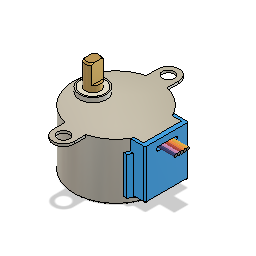
28BYJ-48 (Autodesk Fusion 360 design; units mm, degrees)
Autodesk Fusion 360 part; units mm, degrees
sketch "Sketch1" plane through (0, 0, 0) normal (0, 1, 0) x (1, 0, 0)
  circle A0 centre (0, 0) radius 14
  dimension "d1" = 28
  constraint coincident A0.centre origin
  measures "d1" diameter of A0
extrude "Extrude1" add sketch "Sketch1" along normal blind 19 makes body 1
sketch "Sketch2" plane through (0, 19, 0) normal (0, 1, 0) x (-1, 0, 0)
  circle A0 centre (0, 0) radius 14
  line L0 (14, 0) -> (-15.5, 0)
  line L1 (-15.5, 0) -> (-15.5, -6.3)
  line L2 (-15.5, -6.3) -> (-12.5024, -6.3)
  line L3 (-15.5, 0) -> (-15.5, 6.3)
  line L4 (-15.5, 6.3) -> (-12.5024, 6.3)
  dimension "d4" = 29.5
  dimension "d5" = 6.3
  dimension "d6" = 6.3
  constraint coincident A0 L0.start
  constraint horizontal L0
  constraint perpendicular L0 L1
  constraint coincident A0 L2.end
  constraint perpendicular L1 L2
  constraint perpendicular L0 L3
  constraint coincident A0 L4.end
  constraint perpendicular L3 L4
  measures "d4" distance of L0.start L0.end
  measures "d5" distance of L0.end L1.end
  measures "d6" distance of L0.end L3.end
extrude "Extrude2" add sketch "Sketch2" against normal blind 10 contours A0 L0 L3 L4 | A0 L0 L1 L2 bodies 1
sketch "Sketch3" plane through (0, 19, 0) normal (0, 1, 0) x (-1, 0, 0)
  arc A0 (-12.5024, -6.3) -> (-12.5024, 6.3) centre (0, 0) ccw
  line L0 (-12.5024, 6.3) -> (-15.5, 6.3)
  line L1 (-15.5, 6.3) -> (-15.5, -6.3)
  line L2 (-15.5, -6.3) -> (-12.5024, -6.3)
  line L3 (14, 0) -> (3.2, 0)
  circle A1 centre (7.7, 0) radius 4.5
  circle A2 centre (7.7, 0) radius 4
  dimension "d9" = 10.8
  dimension "d11" = 9
  dimension "d12" = 8
  constraint midpoint A0 L3.start
  constraint horizontal L3
  constraint coincident L3.end A1
  constraint concentric A1 A2
  measures "d9" distance of L3.start L3.end
  measures "d11" diameter of A1
  measures "d12" diameter of A2
extrude "Extrude3" add sketch "Sketch3" along normal blind 1.5 contours L3 A1 A2 | L3 A1 A2 bodies 1
sketch "Sketch4" plane through (0, 19, 0) normal (0, 1, 0) x (-1, 0, 0)
  circle A0 centre (7.7, 0) radius 4
  circle A1 centre (7.7, 0) radius 4
  circle A2 centre (7.7, 0) radius 2.5
  dimension "d15" = 5
  constraint concentric A0 A1
  constraint concentric A1 A2
  measures "d15" diameter of A2
extrude "Extrude4" add sketch "Sketch4" along normal blind 1.5 separate body makes body 2
sketch "Sketch5" plane through (0, 19, 0) normal (0, 1, 0) x (-1, 0, 0)
  circle A0 centre (7.7, 0) radius 4
  circle A1 centre (7.7, 0) radius 2.5
  dimension "d18" = 5
  constraint concentric A0 A1
  measures "d18" diameter of A1
extrude "Extrude5" cut sketch "Sketch5" against normal blind 15 contours A1 bodies 1
extrude "Extrude6" add 1 faces at (-8.3885, 4, -0.2537) along direction (0, 1, 0) blind 24.75 separate body on bodies 1 makes body 3
sketch "Sketch6" plane through (0, 28.75, 0) normal (0, 1, 0) x (-1, 0, 0)
  circle A0 centre (7.7, 0) radius 2.5
  circle A1 centre (7.7, 0) radius 1.5
  line L0 (9.2, 0) -> (9.2, -2)
  line L1 (6.2, 0) -> (6.2, -2)
  line L2 (9.2, 0) -> (9.2, 2)
  line L3 (6.2, 0) -> (6.2, 2)
  dimension "d23" = 3
  constraint concentric A0 A1
  constraint coincident A1 L0.start
  constraint coincident A0 L0.end
  constraint tangent A1 L0
  constraint vertical L0
  constraint coincident A1 L1.start
  constraint coincident A0 L1.end
  constraint tangent A1 L1
  constraint parallel L0 L1
  constraint coincident A0 L2.end
  constraint tangent A1 L2
  constraint coincident A0 L3.end
  constraint tangent A1 L3
  measures "d23" diameter of A1
extrude "Extrude7" cut sketch "Sketch6" against normal blind 6.25 contours A0 L0 L2 | A0 L1 L3 bodies 3
chamfer "Chamfer1" distance 0.5 angle 45 2 edges at (-7.7, 28.75, 2.5) (-7.7, 28.75, -2.5) on bodies 3
sketch "Sketch7" plane through (0, 19, 0) normal (0, 1, 0) x (-1, 0, 0)
  arc A0 (-12.5024, -6.3) -> (-12.5024, 6.3) centre (0, 0) ccw
  line L0 (-12.5024, 6.3) -> (-15.5, 6.3)
  line L1 (-15.5, 6.3) -> (-15.5, -6.3)
  line L2 (-15.5, -6.3) -> (-12.5024, -6.3)
  circle A1 centre (7.7, 0) radius 4.5
  circle A2 centre (0, -17.5) radius 2
  circle A3 centre (0, 17.5) radius 2
  arc A4 (-3.5, -17.5) -> (3.5, -17.5) centre (0, -17.5) ccw
  arc A5 (3.5, 17.5) -> (-3.5, 17.5) centre (0, 17.5) ccw
  line L3 (3.5, -17.5) -> (3.5, -13.5554)
  line L4 (-3.5, -17.5) -> (-3.5, -13.5554)
  line L5 (-3.5, 13.5554) -> (-3.5, 17.5)
  arc A6 (3.5, 13.5554) -> (-3.5, 13.5554) centre (0, 0) ccw
  arc A7 (-3.5, -13.5554) -> (3.5, -13.5554) centre (0, 0) ccw
  line L6 (3.5, 13.5554) -> (3.5, 17.5)
  dimension "d27" = 17.5
  dimension "d28" = 17.5
  dimension "d29" = 4
  dimension "d30" = 4
  dimension "d31" = 7
  dimension "d32" = 7
  constraint concentric A2 A4
  constraint concentric A3 A5
  constraint tangent A5 L3
  constraint vertical L3
  constraint tangent A5 L4
  constraint vertical L4
  constraint coincident A0.centre A6.centre
  constraint coincident A6.start L3
  constraint coincident A0 L4.end
  constraint coincident A0 L5.start
  constraint collinear L4 L5
  constraint concentric A6 A7
  measures "d27" distance of A0.centre A2.centre
  measures "d28" distance of A0.centre A3.centre
  measures "d29" diameter of A2
  measures "d30" diameter of A3
  measures "d31" diameter of A4
  measures "d32" diameter of A5
extrude "Extrude8" add sketch "Sketch7" against normal blind 0.8 contours A0 A4 L3 L4 A7 | A0 A5 L5 A6 L6 bodies 1
fillet "Fillet1" radius 0.5 1 edges at (-13.0526, 0, 5.0626) on bodies 1
sketch "Sketch8" plane through (0, 19, 0) normal (0, 1, 0) x (-1, 0, 0)
  circle A0 centre (0, -17.5) radius 2
  circle A1 centre (0, 17.5) radius 2
  arc A2 (-12.5024, -6.3) -> (-3.5, -13.5554) centre (0, 0) ccw
  line L0 (-3.5, -13.5554) -> (-3.5, -17.5)
  arc A3 (-3.5, -17.5) -> (3.5, -17.5) centre (0, -17.5) ccw
  line L1 (3.5, -17.5) -> (3.5, -13.5554)
  arc A4 (3.5, -13.5554) -> (3.5, 13.5554) centre (0, 0) ccw
  line L2 (3.5, 13.5554) -> (3.5, 17.5)
  arc A5 (3.5, 17.5) -> (-3.5, 17.5) centre (0, 17.5) ccw
  line L3 (-3.5, 17.5) -> (-3.5, 13.5554)
  arc A6 (-3.5, 13.5554) -> (-12.5024, 6.3) centre (0, 0) ccw
  line L4 (-12.5024, 6.3) -> (-15.5, 6.3)
  line L5 (-15.5, 6.3) -> (-15.5, -6.3)
  line L6 (-15.5, -6.3) -> (-12.5024, -6.3)
  circle A7 centre (7.7, 0) radius 4.5
  line L7 (14, 0) -> (-17, 0)
  line L8 (-17, 0) -> (-17, -7.25)
  line L9 (-17, -7.25) -> (-11.9765, -7.25)
  line L10 (-17, 0) -> (-17, 7.25)
  line L11 (-17, 7.25) -> (-11.9765, 7.25)
  dimension "d37" = 7.25
  dimension "d38" = 7.25
  constraint midpoint A4 L7.start
  constraint horizontal L7
  constraint perpendicular L7 L8
  constraint coincident A2 L9.end
  constraint perpendicular L8 L9
  constraint perpendicular L7 L10
  constraint coincident A6 L11.end
  constraint perpendicular L10 L11
  measures "d37" distance of L7.end L8.end
  measures "d38" distance of L7.end L10.end
extrude "Extrude9" add sketch "Sketch8" against normal blind 16.5 separate body contours A2 L5 L6 L7 L8 L9 | A6 L4 L5 L7 L10 L11 makes body 4
sketch "Sketch9" plane through (0, 9, 0) normal (0, -1, 0) x (1, 0, 0)
  line L0 (15.5, -6.3) -> (15.5, 6.3)
  line L1 (15.5, 6.3) -> (12.5024, 6.3)
  arc A0 (12.5024, -6.3) -> (12.5024, 6.3) centre (0, 0) ccw
  line L2 (12.5024, -6.3) -> (15.5, -6.3)
extrude "Extrude10" add sketch "Sketch9" along normal blind 6.5 bodies 4
ref_plane "WorkPlane1" through (14.4883, 15.2, 0) normal (0, 1, 0) x (-1, 0, 0)
sketch "Sketch10" plane through (14.4883, 15.2, 0) normal (0, 1, 0) x (1, 0, 0)
  line L0 (-14.5, 17.5) -> (-14.5, -17.5)
  circle A0 centre (-14.5, 0) radius 15
  line L1 (-14.5, 0) -> (-14.5, 8.625)
  line L2 (-14.5, 8.625) -> (-2.2277, 8.625)
  line L3 (-14.5, 0) -> (-14.5, -8.625)
  line L4 (-14.5, -8.625) -> (-2.2277, -8.625)
  circle A1 centre (-14.5, 0) radius 14
  dimension "d44" = 30
  dimension "d45" = 8.625
  dimension "d46" = 8.625
  dimension "d47" = 28
  constraint vertical L0
  constraint midpoint L0 A0.centre
  constraint coincident A0.centre L1.start
  constraint parallel L0 L1
  constraint coincident A0 L2.end
  constraint perpendicular L1 L2
  constraint perpendicular L2 L3
  constraint coincident A0 L4.end
  constraint perpendicular L0 L4
  constraint concentric A0 A1
  measures "d44" diameter of A0
  measures "d45" distance of A0.centre L1.end
  measures "d46" distance of A0.centre L3.end
  measures "d47" diameter of A1
extrude "Extrude11" add sketch "Sketch10" against normal blind 12.7 contours A0 L2 L4 A1 bodies 4
sketch "Sketch11" plane through (0, 15.2, 0) normal (0, 1, 0) x (-1, 0, 0)
  line L0 (-13.6011, -6.3) -> (-12.5024, -6.3)
  arc A0 (-12.5024, -6.3) -> (-11.9765, -7.25) centre (0, 0) ccw
  line L1 (-11.9765, -7.25) -> (-13.1198, -7.25)
  arc A1 (-13.1198, -7.25) -> (-12.2606, -8.625) centre (0.0117, 0) ccw
  line L2 (-12.2606, -8.625) -> (-11.0159, -8.625)
  arc A2 (-11.0159, 8.625) -> (-11.0159, -8.625) centre (0.0117, 0) ccw
  line L3 (-11.0159, 8.625) -> (-12.2606, 8.625)
  arc A3 (-12.2606, 8.625) -> (-13.1198, 7.25) centre (0.0117, 0) ccw
  line L4 (-13.1198, 7.25) -> (-11.9765, 7.25)
  arc A4 (-11.9765, 7.25) -> (-12.5024, 6.3) centre (0, 0) ccw
  line L5 (-12.5024, 6.3) -> (-13.6011, 6.3)
  arc A5 (-13.6011, 6.3) -> (-13.6011, -6.3) centre (0.0117, 0) ccw
  line L6 (-13.6011, 6.3) -> (-12.5024, 6.3)
  line L7 (-13.6011, -6.3) -> (-12.5024, -6.3)
  line L8 (-12.5024, 6.3) -> (-11.9315, 6.3)
  line L9 (-11.9315, 6.3) -> (-11.9315, -6.3)
  line L10 (-11.9315, -6.3) -> (-12.5024, -6.3)
  constraint coincident L5.end A5.start
  constraint coincident A4.end L5.start
  constraint coincident L0.start A5.end
  constraint coincident L0.end A0.start
  constraint parallel L5 L8
  constraint perpendicular L0 L9
  constraint perpendicular L9 L10
sketch "Sketch12" plane through (0, 19, 0) normal (0, 1, 0) x (-1, 0, 0)
  circle A0 centre (0, -17.5) radius 2
  circle A1 centre (0, 17.5) radius 2
  arc A2 (-12.5024, -6.3) -> (-3.5, -13.5554) centre (0, 0) ccw
  line L0 (-3.5, -13.5554) -> (-3.5, -17.5)
  arc A3 (-3.5, -17.5) -> (3.5, -17.5) centre (0, -17.5) ccw
  line L1 (3.5, -17.5) -> (3.5, -13.5554)
  arc A4 (3.5, -13.5554) -> (3.5, 13.5554) centre (0, 0) ccw
  line L2 (3.5, 13.5554) -> (3.5, 17.5)
  arc A5 (3.5, 17.5) -> (-3.5, 17.5) centre (0, 17.5) ccw
  line L3 (-3.5, 17.5) -> (-3.5, 13.5554)
  arc A6 (-3.5, 13.5554) -> (-12.5024, 6.3) centre (0, 0) ccw
  line L4 (-12.5024, 6.3) -> (-15.5, 6.3)
  line L5 (-15.5, 6.3) -> (-15.5, -6.3)
  line L6 (-15.5, -6.3) -> (-12.5024, -6.3)
  circle A7 centre (7.7, 0) radius 4.5
  circle A8 centre (0, 0) radius 14
  constraint concentric A2 A8
extrude "Extrude12" cut sketch "Sketch12" against normal blind 27 contours A2 A4 A6 A8 bodies 4
extrude "Extrude13" cut sketch "Sketch11" against normal blind 6.15 contours L0 A2 L5 A5 L6 L7 L8 L10 | A2 L8 L9 L10 bodies 4
fillet "Fillet2" radius 0.5 5 edges at (17, 10.75, 7.25) (17, 10.75, -7.25) (15.0599, 2.5, 7.25) (17, 2.5, 0) (15.0599, 2.5, -7.25) on bodies 4
sketch "Sketch13" plane through (17, 0, 0) normal (1, 0, 0) x (0, 0, -1)
  line L0 (-6.75, 19) -> (-6.75, 3)
  line L1 (-6.75, 3) -> (6.75, 3)
  line L2 (6.75, 3) -> (6.75, 19)
  line L3 (6.75, 19) -> (-6.75, 19)
  line L4 (0, 19) -> (0, 17)
  line L5 (0, 17) -> (3.5, 17)
  line L6 (3.5, 17) -> (3.5, 15.75)
  line L7 (3.5, 15.75) -> (-3.5, 15.75)
  line L8 (-3.5, 15.75) -> (-3.5, 17)
  line L9 (-3.5, 17) -> (0, 17)
  dimension "d56" = 2
  dimension "d57" = 3.5
  dimension "d58" = 1.25
  dimension "d59" = 7
  constraint midpoint L3 L4.start
  constraint perpendicular L3 L4
  constraint perpendicular L4 L5
  constraint perpendicular L5 L6
  constraint perpendicular L6 L7
  constraint perpendicular L5 L8
  constraint perpendicular L4 L9
  measures "d56" distance of L4.start L4.end
  measures "d57" distance of L4.end L5.end
  measures "d58" distance of L5.end L6.end
  measures "d59" distance of L6.end L7.end
extrude "Extrude14" cut sketch "Sketch13" against normal blind 5 contours L5 L6 L7 L8 L9 bodies 4
fillet "Fillet3" radius 0.5 4 edges at (16.25, 15.75, -3.5) (16.25, 17, -3.5) (16.25, 17, 3.5) (16.25, 15.75, 3.5) on bodies 4
sketch "Sketch14" plane through (15.5, 0, 0) normal (1, 0, 0) x (0, 0, -1)
  line L0 (6.3, 19) -> (-6.3, 19)
  line L1 (-6.3, 19) -> (-6.3, 9)
  line L2 (-6.3, 9) -> (6.3, 9)
  line L3 (6.3, 9) -> (6.3, 19)
  line L4 (0, 17) -> (0, 16.4)
  circle A0 centre (0, 16.4) radius 0.5
  circle A1 centre (1, 16.4) radius 0.5
  circle A2 centre (2, 16.4) radius 0.5
  circle A3 centre (-1, 16.4) radius 0.5
  circle A4 centre (-2, 16.4) radius 0.5
  dimension "d64" = 0.6
  dimension "d65" = 1
  dimension "d66" = 1
  dimension "d67" = 1
  dimension "d68" = 1
  dimension "d69" = 1
  constraint vertical L4
  constraint coincident L4.end A0.centre
  measures "d64" distance of L4.start L4.end
  measures "d65" diameter of A0
  measures "d66" diameter of A1
  measures "d67" diameter of A2
  measures "d68" diameter of A3
  measures "d69" diameter of A4
extrude "Extrude15" add sketch "Sketch14" along normal blind 6.5 separate body contours A0 | A2 | A1 | A3 | A4 makes body 5
equation "d27 = ( 35 / 2 ) * 1 mm"
equation "d45 = ( 17.25 / 2 ) * 1 mm"
